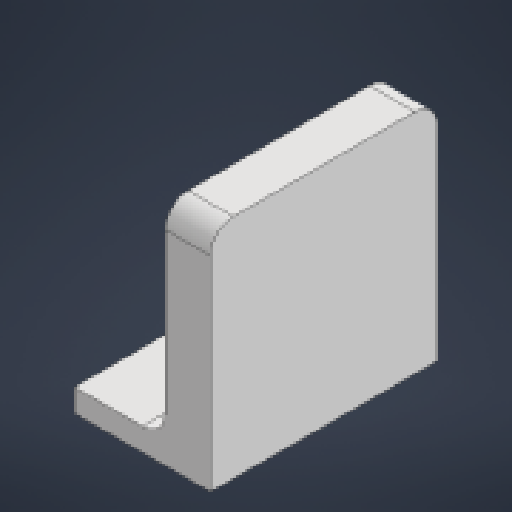
# Autodesk Inventor part: Camera Mount
Saved by Autodesk Inventor 2023 (Build 270158000, 158)
## iProperties
Created: 2023-01-22
Part Number: Camera Mount
Material: Generic
Document SubType Name: Modeling
Designer: Michael
Density: 1 g/cm^3
Appearance: Default
Author: Michael
Autodesk Inventor part; units mm, degrees
ref_plane "YZ Plane" through (0, 0, 0) normal (1, 0, 0) x (0, 1, 0)
ref_plane "XZ Plane" through (0, 0, 0) normal (0, 1, 0) x (-1, 0, 0)
ref_plane "XY Plane" through (0, 0, 0) normal (0, 0, 1) x (1, 0, 0)
sketch "Sketch1" plane through (0, 0, 0) normal (1, 0, 0) x (0, 1, 0)
  line L0 (0, 0) -> (31.75, 0)
  line L1 (31.75, 0) -> (31.75, -31.75)
  line L2 (31.75, -31.75) -> (0, -31.75)
  line L3 (0, -31.75) -> (0, 0)
  dimension "d0" = 31.75
  dimension "d1" = 31.75
  constraints: 8 end point, 2 parallel, 1 horizontal, 1 perpendicular
  measures "d0" distance of L1.end L2.end
  measures "d1" distance of L0.end L1.end
extrude "Extrusion1" add sketch "Sketch1" along normal blind 6.35
sketch "Sketch3" plane through (0, 0, -31.75) normal (0, -1, 0) x (1, 0, 0)
  line L0 (0, 31.75) -> (6.35, 31.75) projected
  line L1 (0, 31.75) -> (-12.7, 31.75)
  line L2 (-12.7, 31.75) -> (-12.7, 0)
  line L3 (-12.7, 0) -> (0, 0)
  line L4 (0, 0) -> (0, 31.75)
  dimension "d10" = 12.7
  constraints: 8 end point, 2 parallel, 1 horizontal, 1 perpendicular
  measures "d10" distance of L3.end L2.end
extrude "Extrusion3" add sketch "Sketch3" against normal blind 3.175
fillet "Fillet1" radius 3.175 1 edges at (0, 3.175, -15.875)
fillet "Fillet2" radius 3.175 2 edges at (3.175, 31.75, -31.75) (3.175, 31.75, 0)
sketch "Sketch4" plane through (0, 3.175, -31.75) normal (0, 1, 0) x (1, 0, 0)
  line L0 (-3.175, 0) -> (-3.175, -31.75) projected
  line L1 (-3.175, 0) -> (-12.7, 0) projected
  line L2 (-12.7, 0) -> (-12.7, -31.75) projected
  line L3 (-12.7, -31.75) -> (-3.175, -31.75) projected
  line L4 (-12.7, -15.875) -> (-3.175, -15.875)
  line L5 (-12.7, -31.75) -> (6.35, -31.75) projected
  line L6 (-7.9375, -31.75) -> (-7.9375, 0)
  point P0 (0, -31.75)
  point P1 (-7.9375, -23.8125)
  point P2 (-7.9375, -7.9375)
  dimension "d15" = 4.7625
  dimension "d17" = 7.9375
  constraints: 4 end point, 3 midpoint, 1 point on line, 1 symmetric about line
  measures "d15" distance from line of L2 point (-7.938, -23.812)
  measures "d17" distance from line of point (-7.938, -23.812) L3
hole "Hole1" at (-7.9375, 3.175, -7.9375) at (-7.9375, 3.175, -23.8125) direction (0, -1, 0) diameter 2.4003 end through all
body "Solid1"
